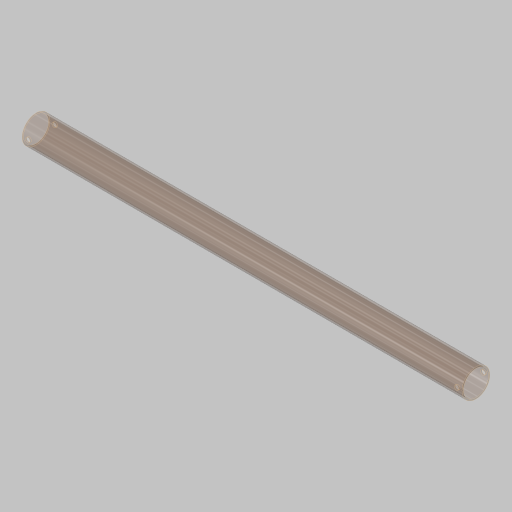
# Autodesk Inventor part: GI - 003
Saved by Autodesk Inventor 2023.5 (Build 275446000, 446)
## iProperties
Created: 2025-01-18
Part Number: GI - 003
Material: Polycarbonate, Smoke
Document SubType Name: Modeling
Designer: mavericks
Density: 1.2 g/cm^3
Appearance: Polycarbonate - Smoked
Mass: 90.9749 g
Surface Area: 959.107 cm^2
Volume: 75.8124 cm^3
Author: mavericks
Autodesk Inventor part; units mm, degrees
ref_plane "YZ Plane" through (0, 0, 0) normal (1, 0, 0) x (0, 1, 0)
ref_plane "XZ Plane" through (0, 0, 0) normal (0, 1, 0) x (-1, 0, 0)
sketch "Sketch1" plane through (0, 0, 0) normal (1, 0, 0) x (0, 1, 0)
  circle A0 centre (0, 0) radius 15.875
  circle A1 centre (0, 0) radius 14.2875
  dimension "d0" = 31.75
  dimension "d2" = 1.5875
  constraints: 2 centre point, 1 coincident
  measures "d0" diameter of A0
  measures "d2" radial gap between concentric circles of A0 A1
extrude "Extrusion1" add sketch "Sketch1" along normal mid plane 500.0625
ref_plane "Work Plane1" through (0, 0, 17.4625) normal (0, 0, 1) x (1, 0, 0)
sketch "Sketch3" plane through (0, 0, 17.4625) normal (0, 0, 1) x (1, 0, 0)
  line L0 (-250.0312, 15.875) -> (-250.0312, -15.875) projected
  line L1 (250.0312, -15.875) -> (250.0312, 15.875) projected
  point P0 (0, 0)
  point P1 (-243.6812, 0)
  point P2 (-250.0312, 0)
  point P3 (243.6812, 0)
  point P4 (250.0312, 0)
  dimension "d15" = 6.35
  dimension "d16" = 6.35
  constraints: 2 horizontal alignment, 2 midpoint
  measures "d15" distance from line of L0 point (-243.681, 0)
  measures "d16" distance from line of L1 point (243.681, 0)
hole "Hole2" at (-243.6812, 0, 17.4625) at (243.6812, 0, 17.4625) direction (0, 0, -1) diameter 5.1054 end through all clearance for "Flat Head Machine Screw (82)" size "#10" standard "Ansi Unified Screw Threads"
body "Solid1"
